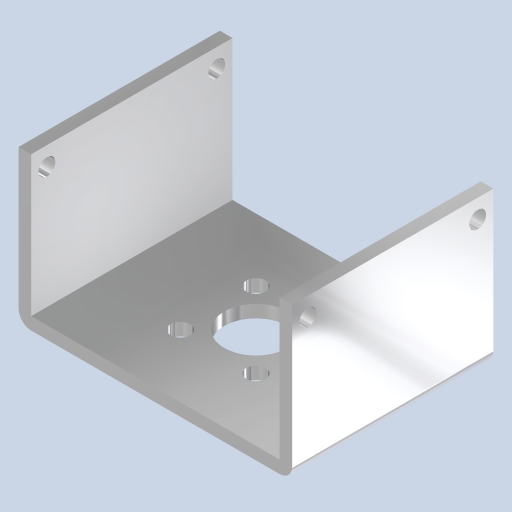
# Autodesk Inventor part: servo_bracket_1170
Saved by Autodesk Inventor 2023 (Build 270158000, 158)
## iProperties
Created: 2015-12-07
Part Number: servo_bracket_1170
Material: アルミニウム 5052
Document SubType Name: シート メタル
Designer: hiroaki
Density: 2.68 g/cm^3
Sheet Metal Rule: Default_mm
Appearance: アルミニウム - フラット
Flat Pattern Width: 3.2 cm
Flat Pattern Length: 8.68637 cm
Flat Pattern Area: 27.7964 cm^2
Sheet Metal Width: 32.000 mm
Sheet Metal Length: 86.864 mm
Sheet Metal Area: 2779.640 mm^2
Mass: 12.622 g
Surface Area: 56.5222 cm^2
Volume: 4.70969 cm^3
Author: hiroaki
Autodesk Inventor part; units mm, degrees
note: some values were not read from the file. Chosen so that the rebuilt part matches the saved one: direction of "穴1".
ref_plane "YZ Plane" through (0, 0, 0) normal (1, 0, 0) x (0, 1, 0)
ref_plane "XZ Plane" through (0, 0, 0) normal (0, 1, 0) x (-1, 0, 0)
ref_plane "XY Plane" through (0, 0, 0) normal (0, 0, 1) x (1, 0, 0)
sketch "スケッチ1" plane through (0, 0, 0) normal (0, 0, 1) x (1, 0, 0)
  line L0 (-19.75, -16) -> (19.75, -16)
  line L1 (19.75, -16) -> (19.75, 16)
  line L2 (19.75, 16) -> (-19.75, 16)
  line L3 (-19.75, 16) -> (-19.75, -16)
  line L4 (-19.75, -16) -> (19.75, 16) construction
  line L5 (19.75, -16) -> (-19.75, 16) construction
  circle A0 centre (0, 0) radius 5.05
  circle A1 centre (-6.0104, 6.0104) radius 1.55
  circle A2 centre (0, 0) radius 8.5 construction
  line L6 (-6.0104, 6.0104) -> (0, 0) construction
  circle A3 centre (-6.0104, -6.0104) radius 1.55
  circle A4 centre (6.0104, -6.0104) radius 1.55
  circle A5 centre (6.0104, 6.0104) radius 1.55
  circle A6 centre (0, 0) radius 8.5
  dimension "d35" = 17
  dimension "d0" = 39.5
  dimension "d1" = 32
  dimension "d2" = 10.1
  dimension "d3" = 3.1
  dimension "d5" = 45
  dimension "d8" = 360
  constraints: 14 end point, 5 centre point, 3 coincident, 2 midpoint, 2 parallel, 1 horizontal, 1 perpendicular, 15 other
  measures "d0" distance of L1.end L2.end
  measures "d1" distance of L2.end L0.start
  measures "d2" diameter of A0
  measures "d3" diameter of A1
  measures "d5" angle of L0 L6
extrude "押し出し1" add sketch "スケッチ1" along normal blind 2 contours L3 L2 L1 L0 | A1 A6 A5 A4 A3
sketch "スケッチ2" plane through (-19.75, -16, 2) normal (-1, 0, 0) x (0, -1, 0)
  line L0 (-32, 0) -> (0, 0)
  line L1 (0, 0) -> (0, 22.3)
  line L2 (0, 22.3) -> (-32, 22.3)
  line L3 (-32, 22.3) -> (-32, 0)
  constraints: 4 end point, 4 other
edge flange "フランジ1" height 22.3 angle 90 thickness 2 bend radius 0.0001 thickness toward (-1, 0, 0) relief tear relief width 2 relief depth 1 corner gap 2 corner form 0 edges at (-19.75, 0, 2) (19.75, 0, 2) wall of the first edge with corners at (-19.75, 16, 2) (-19.75, -16, 2) (-19.75, -16, 24.3) (-19.75, 16, 24.3)
bend "曲げ1"
corner "コーナー1"
sketch "スケッチ4" plane through (21.75, -16, 24.3) normal (1, 0, 0) x (0, 0, -1)
  line L0 (0, 0) -> (0, 32) projected
  line L1 (0, 32) -> (0, 0) construction
  line L2 (0, 16) -> (24.3, 16) construction
  point P0 (3, 2.5)
  point P1 (3, 29.5)
  dimension "d25" = 3
  dimension "d26" = 13.5
  constraints: 2 end point, 1 horizontal, 1 midpoint, 1 symmetric about line, 1 vertical alignment
  measures "d25" distance from line of L0 point (3, 2.5)
  measures "d26" distance from line of L2 point (3, 2.5)
hole "穴1" at (21.75, -13.5, 21.3) at (21.75, 13.5, 21.3) direction (-1, 0, 0) diameter 2.7 end up to surface
mirror "ミラー1" about plane through (0, 0, 0) normal (1, 0, 0) of "穴1"
equation "\"d32\" = Thickness"
equation "\"d12\" = BendReliefWidth"
equation "\"d13\" = BendReliefDepth"
equation "\"d14\" = MinimumRemnant"
equation "\"d15\" = BendRadius"
equation "\"d19\" = CornerReliefSize"
equation "\"d20\" = GapSize"
equation "\"d21\" = JacobiRadiusSize"
equation "\"d34\" = Thickness"
equation "\"BendRadius\" = Thickness"
equation "\"BendReliefWidth\" = Thickness"
equation "\"BendReliefDepth\" = 0.5 * Thickness"
equation "\"CornerReliefSize\" = 4 * Thickness"
equation "\"MinimumRemnant\" = 2 * Thickness"
equation "\"TransitionRadius\" = BendRadius"
equation "\"JacobiRadiusSize\" = BendRadius"
equation "\"GapSize\" = Thickness"
equation "\"Thickness\" = 2"
